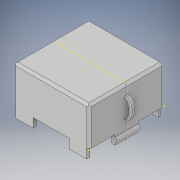
# Autodesk Inventor part: CabeçottaNovo
Saved by Autodesk Inventor 2019.1 (Build 231200000, 200)
## iProperties
Created: 2019-08-01
Part Number: CabeçottaNovo
Material: Genérico
Document SubType Name: Modeling
Designer: IEEE UFABC
Density: 1 g/cm^3
Appearance: Padrão
Author: IEEE UFABC
Autodesk Inventor part; units mm, degrees
ref_plane "YZ Plane" through (0, 0, 0) normal (1, 0, 0) x (0, 1, 0)
ref_plane "XZ Plane" through (0, 0, 0) normal (0, 1, 0) x (-1, 0, 0)
ref_plane "XY Plane" through (0, 0, 0) normal (0, 0, 1) x (1, 0, 0)
sketch "Esboço1" plane through (0, 0, 0) normal (0, 1, 0) x (-1, 0, 0)
  line L0 (0, 0) -> (65, 0)
  line L1 (65, 0) -> (65, -65)
  line L2 (65, -65) -> (0, -65)
  line L3 (0, -65) -> (0, 0)
  line L4 (3, -3) -> (62, -3)
  line L5 (62, -3) -> (62, -62)
  line L6 (62, -62) -> (3, -62)
  line L7 (3, -62) -> (3, -3)
  dimension "d0" = 65
  dimension "d1" = 65
  dimension "d2" = 3
  dimension "d3" = 3
  dimension "d4" = 3
  dimension "d5" = 3
  constraints: 16 end point, 4 parallel, 2 horizontal, 2 perpendicular
  measures "d0" distance of L1.end L2.end
  measures "d1" distance of L0.end L1.end
  measures "d2" distance between parallel lines of L1 L5
  measures "d3" distance between parallel lines of L2 L6
  measures "d4" distance between parallel lines of L3 L7
  measures "d5" distance between parallel lines of L0 L4
extrude "Extrusão1" add sketch "Esboço1" along normal blind 30
sketch "Esboço2" plane through (0, 30, 0) normal (0, 1, 0) x (1, 0, 0)
  line L0 (-65, 65) -> (-65, 0) projected
  line L1 (0, 0) -> (-65, 0)
  line L2 (-65, 0) -> (-65, 65)
  line L3 (-65, 65) -> (0, 65)
  line L4 (0, 65) -> (0, 0)
  constraints: 8 end point, 2 parallel, 1 horizontal, 1 perpendicular
extrude "Extrusão2" add sketch "Esboço2" along normal blind 3
chamfer "Chanfro1" distance 2 angle 45 4 edges at (0, 16.5, -65) (-65, 16.5, -65) (0, 16.5, 0) (-65, 16.5, 0)
chamfer "Chanfro2" distance 2 angle 45 4 edges at (0, 33, -32.5) (-32.5, 33, 0) (-65, 33, -32.5) (-32.5, 33, -65)
sketch "Esboço3" plane through (0, 0, 0) normal (0, -1, 0) x (1, 0, 0)
  point P0 (0, 0)
sketch "Esboço4" plane through (0, 0, 0) normal (0, -1, 0) x (1, 0, 0)
  line L0 (-2, 0) -> (-63, 0) construction
  line L1 (-63, 0) -> (-48, 0)
  line L2 (-48, 0) -> (-48, -3)
  line L3 (-48, -3) -> (-63, -3)
  line L4 (-63, -3) -> (-63, 0)
  line L5 (-2, 0) -> (-17, 0)
  line L6 (-17, 0) -> (-17, -3)
  line L7 (-17, -3) -> (-2, -3)
  line L8 (-2, -3) -> (-2, 0)
  line L9 (-2, -65) -> (-17, -65)
  line L10 (-17, -65) -> (-17, -62)
  line L11 (-17, -62) -> (-2, -62)
  line L12 (-2, -62) -> (-2, -65)
  line L13 (-59, -65) -> (-44, -65)
  line L14 (-44, -65) -> (-44, -62)
  line L15 (-44, -62) -> (-59, -62)
  line L16 (-59, -62) -> (-59, -65)
  point P0 (0, 0)
  dimension "d16" = 15
  dimension "d17" = 15
  constraints: 32 end point, 8 parallel, 4 horizontal, 4 perpendicular, 3 point on line
  measures "d16" distance of L2.end L3.end
  measures "d17" distance of L7.end L6.end
extrude "Extrusão3" add sketch "Esboço4" along normal blind 8
sketch "Esboço5" plane through (0, 0, 0) normal (0, -1, 0) x (1, 0, 0)
  line L0 (-3, -42.5) -> (0, -42.5)
  line L1 (0, -42.5) -> (0, -22.5)
  line L2 (0, -22.5) -> (-3, -22.5)
  line L3 (-3, -22.5) -> (-3, -42.5)
  line L4 (-62, -42.5) -> (-65, -42.5)
  line L5 (-65, -42.5) -> (-65, -22.5)
  line L6 (-65, -22.5) -> (-62, -22.5)
  line L7 (-62, -22.5) -> (-62, -42.5)
  point P0 (0, 0)
  constraints: 16 end point, 4 parallel, 2 horizontal, 2 perpendicular
extrude "Extrusão4" add sketch "Esboço5" along normal blind 8
sketch "Esboço6" plane through (-62, 0, -42.5) normal (0, 0, -1) x (-1, 0, 0)
  line L0 (-62, 0) -> (-62, -8) projected
  ellipse E0 centre (-62, -4) end of major axis (-62, -6) minor radius 1.8 (-62, -2) -> (-62, -6) ccw
  line L1 (3, 0) -> (3, -8) projected
  ellipse E1 centre (3, -4) end of major axis (3, -6) minor radius 1.8 (3, -6) -> (3, -2) ccw
  dimension "d24" = 2
  dimension "d25" = 1.8
  dimension "d26" = 1.8
  constraints: 4 point on line, 2 midpoint, 8 other
extrude "Extrusão5" add sketch "Esboço6" against normal blind 20
sketch "Esboço7" plane through (-2, 31, -65) normal (0, 0, -1) x (-1, 0, 0)
  line L0 (15, -31) -> (42, -31) construction
  line L1 (61, 0) -> (0, 0) construction
  line L2 (0, -31) -> (0, 0) construction
  circle A0 centre (14.25, -16.4194) radius 8.5
  circle A1 centre (46.75, -16.4194) radius 8.5
  line L3 (61, 0) -> (61, -31) construction
  line L4 (42, -31) -> (15, -31) projected
  point P0 (-2, -31)
  dimension "d29" = 17
  dimension "d30" = 17
  dimension "d31" = 14.25
  dimension "d32" = 14.25
  constraints: 2 centre point, 2 end point, 1 vertical
  measures "d29" diameter of A0
  measures "d30" diameter of A1
  measures "d31" distance from line of L2 A0.centre
  measures "d32" distance from line of A1.centre L3
extrude "Extrusão6" cut sketch "Esboço7" against normal blind 8
sketch "Esboço8" plane through (-2, 31, -65) normal (0, 0, -1) x (-1, 0, 0)
  circle A0 centre (14.25, -16.4194) radius 8.5 projected
  line L0 (14.25, -16.4194) -> (14.25, -24.9194) construction
  circle A1 centre (46.75, -16.4194) radius 8.5 projected
  line L1 (46.75, -16.4194) -> (46.75, -24.9194) construction
  line L2 (14.25, -24.9194) -> (46.75, -24.9194) construction
  line L3 (46.75, -20.6694) -> (36.8683, -20.6694) construction
  line L4 (36.8683, -20.6694) -> (36.8683, -24.9194) construction
  circle A2 centre (28.5, -21.875) radius 2.125
  point P0 (-2, -31)
  constraints: 10 end point, 2 perpendicular, 2 vertical alignment, 1 centre point, 1 horizontal, 1 midpoint, 1 parallel, 1 point on line, 1 vertical, 2 other
extrude "Extrusão7" add sketch "Esboço8" along normal blind 2 contours A2
fillet "Arredondamento1" radius 2 1 edges at (-28.375, 9.125, -67)
ref_plane "Plano de trabalho1" through (-2, 31, -32.5) normal (0, 0, -1) x (-1, 0, 0)
sketch "Esboço9" plane through (-2, 31, -32.5) normal (0, 0, -1) x (-1, 0, 0)
  line L0 (-2, 0) -> (-2, -31) projected
  line L1 (-2, -31) -> (-2, 0) construction
  line L2 (1, -31) -> (1, -1) construction
  line L3 (63, -31) -> (63, 0) projected
  ellipse E0 centre (63, -15.5) end of major axis (63, -6.5) minor radius 6 (63, -24.5) -> (63, -6.5) ccw
  ellipse E1 centre (-2, -15.5) end of major axis (-2, -6.5) minor radius 6 (-2, -6.5) -> (-2, -24.5) ccw
  ellipse E2 centre (-2, -15.5) end of major axis (-2, -6.5) minor radius 6 (0.2775, -23.8264) -> (1, -23.2942) ccw
  ellipse E3 centre (63, -15.5) end of major axis (63, -8.2142) minor radius 4 (63, -22.7858) -> (63, -8.2142) ccw
  line L4 (0.2775, -36.0298) -> (0.2775, -23.8264) construction
  line L5 (0.2775, -21.4895) -> (0.2775, -15.5) construction
  ellipse E4 centre (-2, -15.5) end of major axis (-2, -8.2142) minor radius 4 (-2, -8.2142) -> (-2, -22.7858) ccw
  ellipse E5 centre (-2, -15.5) end of major axis (-2, -8.2142) minor radius 4 (0.2775, -21.4895) -> (1, -20.3191) ccw
  line L6 (-2, -6.5) -> (-2, -24.5)
  line L7 (-2, -6.5) -> (-2, -24.5)
  line L8 (-2, -8.2142) -> (-2, -6.5)
  line L9 (-2, -22.7858) -> (-2, -24.5)
  dimension "d41" = 6
  dimension "d43" = 4
  constraints: 14 end point, 10 point on line, 4 collinear, 2 coincident, 2 midpoint, 2 parallel, 1 vertical, 24 other
extrude "Extrusão8" add sketch "Esboço9" along normal mid plane 4 contours L0 E4 E1 | L3 E3 E0
fillet "Arredondamento2" radius 1 2 edges at (-71, 15.5, -30.5) (-71, 15.5, -34.5)
fillet "Arredondamento3" radius 1 2 edges at (6, 15.5, -34.5) (6, 15.5, -30.5)
sketch "Esboço10" plane through (-2, 31, -65) normal (0, 0, -1) x (-1, 0, 0)
  point P0 (-2, -31)
sketch "Esboço11" plane through (-2, 31, -65) normal (0, 0, -1) x (-1, 0, 0)
  point P0 (-2, -31)
sketch "Esboço12" plane through (-2, 0, -62) normal (1, 0, 0) x (0, 0, -1)
  line L0 (0, -8) -> (3, -8) projected
  line L1 (3.2206, 0) -> (1.5, 0)
  line L2 (1.5, 0) -> (1.5, -8)
  line L3 (1.5, -8) -> (3.2206, -8)
  line L4 (3.2206, -8) -> (3.2206, 0)
  point P0 (-62, 0)
  constraints: 8 end point, 2 parallel, 1 horizontal, 1 midpoint, 1 perpendicular
extrude "Extrusão9" cut sketch "Esboço12" against normal blind 69
sketch "Esboço13" plane through (-2, 0, -65) normal (0, 0, -1) x (-1, 0, 0)
  point P0 (-2, 0)
